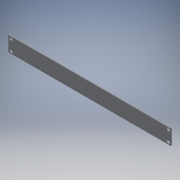
# Autodesk Inventor part: 1U 19pol 3mm painel
Saved by Autodesk Inventor 2016 (Build 200138000, 138)
## iProperties
Created: 2015-01-27
Part Number: 1U 19pol 3mm painel
Material: Genérico
Document SubType Name: Modeling
Designer: fernando.santanna
Density: 1 g/cm^3
Appearance: Default
Author: fernando.santanna
Autodesk Inventor part; units mm, degrees
ref_plane "YZ Plane" through (0, 0, 0) normal (1, 0, 0) x (0, 1, 0)
ref_plane "XZ Plane" through (0, 0, 0) normal (0, 1, 0) x (-1, 0, 0)
ref_plane "XY Plane" through (0, 0, 0) normal (0, 0, 1) x (1, 0, 0)
sketch "Esboço1" plane through (0, 0, 0) normal (0, 1, 0) x (-1, 0, 0)
  line L0 (0, 0) -> (-479, 0)
  line L1 (-479, 0) -> (-479, 44.5)
  line L2 (-479, 44.5) -> (0, 44.5)
  line L3 (0, 44.5) -> (0, 0)
  dimension "d0" = 479
  dimension "d1" = 44.5
  constraints: 8 end point, 2 parallel, 1 horizontal, 1 perpendicular
  measures "d0" distance of L1.end L2.end
  measures "d1" distance of L0.end L1.end
extrude "Extrusão1" add sketch "Esboço1" along normal blind 3
sketch "Esboço2" plane through (0, 3, 0) normal (0, 1, 0) x (1, 0, 0)
  line L0 (479, 0) -> (0, 0) projected
  line L1 (0, 0) -> (0, -44.5) projected
  line L2 (5.25, -3) -> (10.75, -3)
  line L3 (13.5, -3) -> (13.5, -10)
  line L4 (13.5, -10) -> (2.5, -10)
  line L5 (2.5, -10) -> (2.5, -3)
  arc A0 (5.25, -3) -> (5.25, -10) centre (6.1023, -6.5) ccw
  arc A1 (10.75, -10) -> (10.75, -3) centre (9.8977, -6.5) ccw
  line L6 (10.75, -3) -> (10.75, -10) construction
  line L7 (10.75, -3) -> (17.75, -3) construction
  dimension "d8" = 7
  dimension "d10" = 11
  dimension "d11" = 2.5
  dimension "d12" = 3
  dimension "d13" = 90
  dimension "d14" = 5.5
  dimension "d20" = 3.6023
  dimension "d21" = 3.6023
  constraints: 12 end point, 4 point on circle, 2 centre point, 2 horizontal, 2 parallel, 2 perpendicular, 2 point on line, 2 tangent, 1 horizontal alignment
  measures "d8" distance of L3.start L3.end
  measures "d10" distance of L3.end L4.end
  measures "d11" distance between parallel lines of L5 L1
  measures "d12" distance between parallel lines of L0 L2
  measures "d13" angle of L6 L7
  measures "d14" distance of L2.start L2.end
  measures "d20" distance from line of L5 A0.centre
  measures "d21" distance from line of L3 A1.centre
extrude "Extrusão2" cut sketch "Esboço2" against normal blind 10 contours L2 A1 L4 A0
pattern_linear "Padrão retangular1" count 2 spacing 31.5 along (0, 0, 1) count 2 spacing 463 along (1, 0, 0) of "Extrusão2"
equation "\"d20\" = d21"
